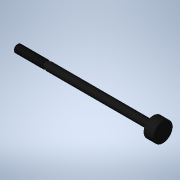
# Autodesk Inventor part: CJ2D10-30Z_ROD
Saved by Autodesk Inventor 2021 (Build 250183000, 183)
## iProperties
Created: 2025-12-04
Part Number: CJ2D10-30Z_ROD
Material: Generic
Catalog Web Link: www.3dfindit.com
Description: CJ2-Z ROD-Air Cylinder/Standard: Double Acting Single Rod
Vendor: SMC
Document SubType Name: Modeling
Designer: psAdmin
Manufacturer: SMC
Mass: 1.27153 g
Surface Area: 12.0141 cm^2
Volume: 1.27153 cm^3
Density: 1 g/cm^3
Appearance: PSOLRGB-128-128-128
Category: PARTsolutions
Company: SMC
Title: CJ2D10-30Z_ROD
Author: Cadenas PARTsolutions
Comments: Air Cylinder/Standard: Double Acting Single Rod
PSOL_IDENT_0: {$CADENAS_DATA/23d-libs/smc_jp/actuator/standard_air_cylinder/cj2/cj2_z/parts/cj2_z_rod.prj},197 {VT
PSOL_IDENT_1: YP=3D},{NB=CJ2D10-30Z_ROD},{LINA=CJ2D10-30Z_ROD},{NN=CJ2-Z ROD},{DATE=02.12.2025 09:45:30},{GEOMDATE=
PSOL_IDENT_2: 08.08.2023 07:41:00},{VERSION=},{LINEID=400},{WBVAR=STROKE,CUSHION,RODB},{WBNUMERIC=STROKE}  {NB=CJ2
PSOL_IDENT_3: D10-30Z_ROD},{LINA=CJ2D10-30Z_ROD},{KT=DUMMY},{ORDER=CJ2D10-30Z},{BORE=10},{MOUNT=(D) Double clevis}
PSOL_IDENT_4: ,{MOUNTX=D},{STROKE=30},{CUSHION=},{RODB=},{A=15},{D=4},{H=28},{MM=M4x0.7},{MM1=4},{MM2=0.7},{NA=12.
PSOL_IDENT_5: 5},{NA1=12.5},{NA2=21.000},{S=46},{S1=46.000},{S2=65.000},{NB1=22.500},{SMAX=400.000},{P=8},{P1=8.00
PSOL_IDENT_6: 0},{P2=8.000},{P3=8.000}
NB: CJ2D10-30Z_ROD
NN: CJ2-Z ROD
NT: Air Cylinder/Standard: Double Acting Single Rod
NBSYN: $ORDER._ROD
LINA: CJ2D10-30Z_ROD
CATALOG: SMC (JP
BORE: 10
MOUNT: (D) Double clevis
STROKE: 30
CUSHION: (-) Rubber cushion
RODB: (-) None
A: 15
D: 4
H: 28
MM: M4x0.7
MM1: 4
MM2: 0.7
NA1: 12.5
NA2: 21
S1: 46
S2: 65
NB1: 22.5
SMAX: 400
P1: 8
P2: 8
P3: 8
SUPPLIER: SMC
ARTICLENO: CJ2D10-30Z_ROD
BOMINFO: CJ2D10-30Z_ROD
CREATOR: CADENAS GmbH
Autodesk Inventor part; units mm, degrees
sketch "Sketch_2" plane through (0, 0, 0) normal (0, 0, 1) x (1, 0, 0)
  line L0 (75.5, 0) -> (0, 0)
  line L1 (0, 0) -> (0, 1.5705)
  line L2 (0, 1.5705) -> (0.4295, 2)
  line L3 (0.4295, 2) -> (15, 2)
  line L4 (15, 2) -> (15, 1.65)
  line L5 (15, 1.65) -> (16.5, 1.65)
  line L6 (16.5, 1.65) -> (16.5, 2)
  line L7 (16.5, 2) -> (70.5, 2)
  line L8 (70.5, 2) -> (70.5, 5)
  line L9 (70.5, 5) -> (75.5, 5)
  line L10 (75.5, 5) -> (75.5, 0)
  line L11 (75.5, 0) -> (0, 0)
  constraints: 24 end point
revolve "Revolution1" add sketch "Sketch_2" angle 360 about axis through (75.5, 0, 0) along (1, 0, 0)
thread "Thread1" size "M4x0.7" class "6g" standard "ISO Metric profile" full length
ref_plane "ROD_BA_XY" through (8, 0, 0) normal (-1, 0, 0) x (0, 0, -1)
ref_plane "ROD_BA_YZ" through (8, 0, 0) normal (0, 0, -1) x (0, -1, 0)
ref_plane "ROD_BA_ZX" through (8, 0, 0) normal (0, -1, 0) x (-1, 0, 0)
ref_plane "ROD_BODY_XY" through (28, 0, 0) normal (1, 0, 0) x (0, 0, -1)
ref_plane "ROD_BODY_YZ" through (28, 0, 0) normal (0, 0, -1) x (0, 1, 0)
ref_plane "ROD_BODY_ZX" through (28, 0, 0) normal (0, 1, 0) x (1, 0, 0)
ref_plane "rodnt1_XY" through (7.5, 0, 0) normal (1, 0, 0) x (0, 0, -1)
ref_plane "rodnt1_YZ" through (7.5, 0, 0) normal (0, 0, -1) x (0, 1, 0)
ref_plane "rodnt1_ZX" through (7.5, 0, 0) normal (0, 1, 0) x (1, 0, 0)
body "Solid1"
